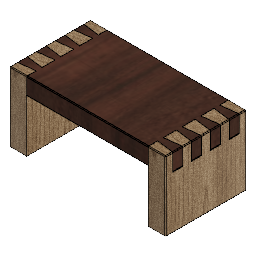
one-step-stool-dovetail (Autodesk Fusion 360 design; units mm, degrees)
Autodesk Fusion 360 part; units mm, degrees
sketch "Sketch1" plane through (0, 0, 0) normal (0, 0, 1) x (1, 0, 0) in component "Top"
  line L0 (38.1, 184.15) -> (38.1, 0) construction
  line L1 (342.9, 92.075) -> (0, 92.075) construction
  line L2 (38.1, 92.075) -> (38.1, 74.6294)
  line L3 (38.1, 74.6294) -> (0, 79.375)
  line L4 (0, 79.375) -> (0, 57.15)
  line L5 (0, 57.15) -> (38.1, 61.8956)
  line L6 (38.1, 61.8956) -> (38.1, 33.3544)
  line L7 (38.1, 33.3544) -> (0, 38.1)
  line L8 (0, 38.1) -> (0, 15.875)
  line L9 (0, 15.875) -> (38.1, 20.6206)
  line L10 (38.1, 20.6206) -> (38.1, 0)
  line L11 (0, 92.075) -> (0, 0) construction
  line L12 (38.1, 163.5294) -> (38.1, 184.15)
  line L13 (0, 168.275) -> (38.1, 163.5294)
  line L14 (0, 146.05) -> (0, 168.275)
  line L15 (38.1, 150.7956) -> (0, 146.05)
  line L16 (38.1, 122.2544) -> (38.1, 150.7956)
  line L17 (0, 127) -> (38.1, 122.2544)
  line L18 (0, 104.775) -> (0, 127)
  line L19 (38.1, 109.5206) -> (0, 104.775)
  line L20 (38.1, 92.075) -> (38.1, 109.5206)
  line L21 (171.45, 0) -> (171.45, 398.9045) construction
  line L22 (342.9, 104.775) -> (342.9, 127)
  line L23 (304.8, 92.075) -> (304.8, 109.5206)
  line L24 (342.9, 15.875) -> (304.8, 20.6206)
  line L25 (304.8, 109.5206) -> (342.9, 104.775)
  line L26 (342.9, 127) -> (304.8, 122.2544)
  line L27 (304.8, 163.5294) -> (304.8, 184.15)
  line L28 (304.8, 74.6294) -> (342.9, 79.375)
  line L29 (304.8, 92.075) -> (304.8, 74.6294)
  line L30 (304.8, 122.2544) -> (304.8, 150.7956)
  line L31 (342.9, 168.275) -> (304.8, 163.5294)
  line L32 (304.8, 33.3544) -> (342.9, 38.1)
  line L33 (304.8, 184.15) -> (304.8, 0) construction
  line L34 (304.8, 20.6206) -> (304.8, 0)
  line L35 (304.8, 61.8956) -> (304.8, 33.3544)
  line L36 (342.9, 92.075) -> (342.9, 0) construction
  line L37 (342.9, 146.05) -> (342.9, 168.275)
  line L38 (342.9, 79.375) -> (342.9, 57.15)
  line L39 (304.8, 150.7956) -> (342.9, 146.05)
  line L40 (342.9, 38.1) -> (342.9, 15.875)
  line L41 (342.9, 57.15) -> (304.8, 61.8956)
  line L42 (38.1, 184.15) -> (304.8, 184.15)
  line L43 (38.1, 0) -> (304.8, 0)
  point P0 (342.9, 0)
  dimension "d5" = 38.1
  dimension "d6" = 82.9
  dimension "d8" = 82.9
  dimension "d9" = 82.9
  dimension "d10" = 82.9
  dimension "d11" = 12.7
  dimension "d12" = 22.225
  dimension "d13" = 15.875
  dimension "d14" = 22.225
  dimension "d15" = 92.075
  dimension "d16" = 342.9
  dimension "d17" = 184.15
  constraint coincident L11.end origin
  constraint midpoint L0 L2.start
  constraint coincident L0 L2.end
  constraint coincident L0 L5.end
  constraint coincident L0 L6.end
  constraint parallel L0 L6
  constraint coincident L0 L9.end
  constraint vertical L4
  constraint vertical L8
  constraint collinear L8 L11
  constraint collinear L4 L11
  constraint symmetric L0.end L1 L0.start
  constraint symmetric L1 L2.start L20.start
  constraint symmetric L1 L2.end L19.start
  constraint symmetric L1 L3.end L18.start
  constraint symmetric L1 L4.end L17.start
  constraint symmetric L1 L5.end L16.start
  constraint symmetric L1 L6.end L15.start
  constraint symmetric L1 L7.end L14.start
  constraint symmetric L1 L8.end L13.start
  constraint symmetric L1 L9.end L12.start
  constraint symmetric L11.end L21 L36.end
  constraint symmetric L11.end L21 P0
  constraint symmetric L0.start L21 L27.end
  constraint symmetric L0.end L21 L33.end
  constraint symmetric L1.end L21 L1.start
  constraint symmetric L2.start L21 L23.start
  constraint symmetric L2.end L21 L28.start
  constraint symmetric L3.end L21 L28.end
  constraint symmetric L4.end L21 L38.end
  constraint symmetric L5.end L21 L35.start
  constraint symmetric L6.end L21 L32.start
  constraint symmetric L7.end L21 L32.end
  constraint symmetric L8.end L21 L24.start
  constraint symmetric L9.end L21 L24.end
  constraint symmetric L12.start L21 L27.start
  constraint symmetric L13.start L21 L31.start
  constraint symmetric L14.start L21 L37.start
  constraint symmetric L15.start L21 L30.end
  constraint symmetric L16.start L21 L26.end
  constraint symmetric L17.start L21 L22.end
  constraint symmetric L18.start L21 L22.start
  constraint symmetric L19.start L21 L23.end
  constraint perpendicular L27 L42
  constraint perpendicular L33 L43
  measures "d5" distance of L11.end L0.end
  measures "d6" angle of L2 L3
  measures "d8" angle of L5 L6
  measures "d9" angle of L6 L7
  measures "d10" angle of L9 L10
  measures "d11" distance of L1.end L3.end
  measures "d12" distance of L3.end L4.end
  measures "d13" distance of L11.end L8.end
  measures "d14" distance of L7.end L8.end
  measures "d15" distance of L11.end L1.end
  measures "d16" distance of L14 L37
  measures "d17" distance of L42 L43
sketch "Sketch2" plane through (0, 0, 0) normal (0, 0, 1) x (1, 0, 0) in component "Top"
  line L0 (3.0624, 88.9) -> (129.9288, 88.9) construction
  line L1 (38.1, 0) -> (38.1, 20.6206)
  line L2 (38.1, 20.6206) -> (0, 15.875)
  line L3 (0, 15.875) -> (0, 38.1)
  line L4 (0, 38.1) -> (38.1, 33.3544)
  line L5 (38.1, 33.3544) -> (38.1, 61.8956)
  line L6 (38.1, 61.8956) -> (0, 57.15)
  line L7 (0, 57.15) -> (0, 79.375)
  line L8 (0, 79.375) -> (38.1, 74.6294)
  line L9 (38.1, 74.6294) -> (38.1, 88.9)
  line L10 (38.1, 61.8956) -> (38.1, 74.6294) construction
  line L11 (0, 0) -> (101.4226, 0) construction
  line L12 (0, 0) -> (0, 254.7903) construction
  line L13 (38.1, 177.8) -> (38.1, 157.1794)
  line L14 (38.1, 157.1794) -> (0, 161.925)
  line L15 (0, 161.925) -> (0, 139.7)
  line L16 (0, 139.7) -> (38.1, 144.4456)
  line L17 (38.1, 144.4456) -> (38.1, 115.9044)
  line L18 (38.1, 115.9044) -> (0, 120.65)
  line L19 (0, 120.65) -> (0, 98.425)
  line L20 (0, 98.425) -> (38.1, 103.1706)
  line L21 (38.1, 103.1706) -> (38.1, 88.9)
  line L22 (171.45, -19.8765) -> (171.45, 334.6379) construction
  line L23 (304.8, 61.8956) -> (304.8, 74.6294) construction
  line L24 (304.8, 74.6294) -> (304.8, 88.9)
  line L25 (342.9, 38.1) -> (304.8, 33.3544)
  line L26 (342.9, 79.375) -> (304.8, 74.6294)
  line L27 (304.8, 0) -> (304.8, 20.6206)
  line L28 (342.9, 120.65) -> (342.9, 98.425)
  line L29 (304.8, 20.6206) -> (342.9, 15.875)
  line L30 (342.9, 161.925) -> (342.9, 139.7)
  line L31 (342.9, 139.7) -> (304.8, 144.4456)
  line L32 (304.8, 33.3544) -> (304.8, 61.8956)
  line L33 (304.8, 177.8) -> (304.8, 157.1794)
  line L34 (304.8, 103.1706) -> (304.8, 88.9)
  line L35 (304.8, 157.1794) -> (342.9, 161.925)
  line L36 (304.8, 115.9044) -> (342.9, 120.65)
  line L37 (342.9, 15.875) -> (342.9, 38.1)
  line L38 (342.9, 98.425) -> (304.8, 103.1706)
  line L39 (304.8, 144.4456) -> (304.8, 115.9044)
  line L40 (342.9, 57.15) -> (342.9, 79.375)
  line L41 (304.8, 61.8956) -> (342.9, 57.15)
  line L42 (38.1, 0) -> (304.8, 0)
  line L43 (38.1, 177.8) -> (304.8, 177.8)
  line L44 (342.9, 177.8) -> (0, 177.8)
  line L45 (0, 177.8) -> (0, 0)
  line L46 (0, 0) -> (342.9, 0)
  line L47 (342.9, 0) -> (342.9, 177.8)
  line L48 (0, 177.8) -> (0, 0)
  line L49 (38.1, 177.8) -> (38.1, 0)
  point P0 (342.9, 0)
  point P1 (339.8376, 88.9)
  point P2 (342.9, 0)
  point P3 (342.9, 0)
  dimension "d21" = 88.9
  dimension "d22" = 38.1
  dimension "d24" = 82.9
  dimension "d25" = 38.1
  dimension "d26" = 97.1
  dimension "d27" = 9.525
  dimension "d28" = 15.875
  dimension "d30" = 22.225
  dimension "d31" = 22.225
  dimension "d32" = 171.45
  constraint vertical L1
  constraint parallel L1 L3
  constraint parallel L4 L8
  constraint perpendicular L0 L9
  constraint parallel L2 L6
  constraint coincident L0 L9.end
  constraint coincident L11.start L12.start
  constraint perpendicular L3 L11
  constraint coincident L1.start L11
  constraint collinear L5 L9
  constraint collinear L1 L5
  constraint perpendicular L11 L12
  constraint collinear L7 L12
  constraint symmetric L0 L1.start L13.start
  constraint symmetric L0 L1.end L13.end
  constraint symmetric L0 L2.end L14.end
  constraint symmetric L0 L3.end L15.end
  constraint symmetric L0 L4.end L16.end
  constraint symmetric L0 L5.end L17.end
  constraint symmetric L0 L6.end L18.end
  constraint symmetric L0 L7.end L19.end
  constraint symmetric L0 L8.end L20.end
  constraint symmetric L0 L9.end L21.end
  constraint vertical L22
  constraint symmetric L11.start L22 P3
  constraint symmetric L0.start L22 P1
  constraint symmetric L1.start L22 L27.start
  constraint symmetric L1.end L22 L27.end
  constraint symmetric L2.end L22 L29.end
  constraint symmetric L3.end L22 L25.start
  constraint symmetric L4.end L22 L25.end
  constraint symmetric L5.end L22 L23.start
  constraint symmetric L6.end L22 L40.start
  constraint symmetric L7.end L22 L26.start
  constraint symmetric L8.end L22 L23.end
  constraint symmetric L9.end L22 L24.end
  constraint symmetric L13.start L22 L33.start
  constraint symmetric L13.end L22 L33.end
  constraint symmetric L14.end L22 L30.start
  constraint symmetric L15.end L22 L30.end
  constraint symmetric L16.end L22 L31.end
  constraint symmetric L17.end L22 L36.start
  constraint symmetric L18.end L22 L28.start
  constraint symmetric L19.end L22 L28.end
  constraint symmetric L20.end L22 L34.start
  constraint horizontal L44
  constraint vertical L45
  constraint horizontal L46
  constraint vertical L47
  constraint collinear L42 L46
  constraint collinear L15 L45
  constraint collinear L37 L47
  constraint collinear L43 L44
  measures "d21" vertical distance of L11.start L0.start
  measures "d22" distance of L1 L3
  measures "d24" angle of L8 L9
  measures "d25" horizontal distance of L7.end L9.end
  measures "d26" angle of L6 L10
  measures "d27" distance of L0 L7.end
  measures "d28" distance of L2.end L11
  measures "d30" distance of L6.end L7.end
  measures "d31" distance of L2.end L3.end
  measures "d32" distance of L12 L22
sketch "Sketch3" plane through (0, 0, 0) normal (0, 0, 1) x (1, 0, 0) in component "Top"
  line L0 (342.9, 177.8) -> (0, 177.8)
  line L1 (0, 177.8) -> (0, 0)
  line L2 (0, 0) -> (342.9, 0)
  line L3 (342.9, 0) -> (342.9, 177.8)
  dimension "d33" = 177.8
  dimension "d34" = 342.9
  constraint horizontal L0
  constraint vertical L1
  constraint horizontal L2
  constraint vertical L3
  constraint coincident L1.end L2.start
  measures "d33" distance of L0.start L2.end
  measures "d34" distance of L1.end L2.end
extrude "Extrude1" add sketch "Sketch3" along normal blind 38.1 makes body 1 in component "Top"
sketch "Sketch4" plane through (0, 0, 38.1) normal (0, 0, 1) x (-1, 0, 0) in component "Top"
  line L0 (-342.9, 0) -> (-342.9, -177.8)
  line L1 (-342.9, -177.8) -> (0, -177.8)
  line L2 (0, -177.8) -> (0, 0)
  line L3 (0, 0) -> (-342.9, 0)
  line L4 (0, -88.9) -> (-342.9, -88.9) construction
  line L5 (-171.45, -177.8) -> (-171.45, 0)
  line L6 (-38.1, -177.8) -> (-38.1, 0) construction
  line L7 (-38.1, -88.9) -> (-38.1, -74.6294)
  line L8 (-38.1, -74.6294) -> (0, -79.375)
  line L9 (0, -79.375) -> (0, -57.15)
  line L10 (0, -57.15) -> (-38.1, -61.8956)
  line L11 (-38.1, -61.8956) -> (-38.1, -33.3544)
  line L12 (-38.1, -33.3544) -> (0, -38.1)
  line L13 (0, -38.1) -> (0, -15.875)
  line L14 (0, -15.875) -> (-38.1, -20.6206)
  line L15 (-38.1, -20.6206) -> (-38.1, 0)
  line L16 (-38.1, -157.1794) -> (-38.1, -177.8)
  line L17 (0, -161.925) -> (-38.1, -157.1794)
  line L18 (0, -139.7) -> (0, -161.925)
  line L19 (-38.1, -144.4456) -> (0, -139.7)
  line L20 (-38.1, -115.9044) -> (-38.1, -144.4456)
  line L21 (0, -120.65) -> (-38.1, -115.9044)
  line L22 (0, -98.425) -> (0, -120.65)
  line L23 (-38.1, -103.1706) -> (0, -98.425)
  line L24 (-38.1, -88.9) -> (-38.1, -103.1706)
  line L25 (-304.8, -177.8) -> (-304.8, 0) construction
  line L26 (-342.9, -161.925) -> (-304.8, -157.1794)
  line L27 (-342.9, -139.7) -> (-342.9, -161.925)
  line L28 (-304.8, -144.4456) -> (-342.9, -139.7)
  line L29 (-304.8, -115.9044) -> (-304.8, -144.4456)
  line L30 (-342.9, -120.65) -> (-304.8, -115.9044)
  line L31 (-342.9, -98.425) -> (-342.9, -120.65)
  line L32 (-304.8, -103.1706) -> (-342.9, -98.425)
  line L33 (-304.8, -88.9) -> (-304.8, -103.1706)
  line L34 (-304.8, -74.6294) -> (-342.9, -79.375)
  line L35 (-342.9, -79.375) -> (-342.9, -57.15)
  line L36 (-342.9, -57.15) -> (-304.8, -61.8956)
  line L37 (-304.8, -61.8956) -> (-304.8, -33.3544)
  line L38 (-304.8, -33.3544) -> (-342.9, -38.1)
  line L39 (-342.9, -38.1) -> (-342.9, -15.875)
  line L40 (-342.9, -15.875) -> (-304.8, -20.6206)
  line L41 (-304.8, -20.6206) -> (-304.8, 0)
  line L42 (-304.8, -157.1794) -> (-304.8, -177.8)
  line L43 (-304.8, -103.1706) -> (-304.8, -74.6294)
  point P0 (-38.1, -88.9)
  dimension "d37" = 38.1
  dimension "d38" = 38.1
  dimension "d40" = 82.9
  dimension "d41" = 9.525
  dimension "d42" = 88.9
  dimension "d43" = 22.225
  dimension "d44" = 82.9
  dimension "d45" = 82.9
  dimension "d46" = 82.9
  dimension "d47" = 22.225
  dimension "d48" = 15.875
  constraint midpoint L2 L4.start
  constraint midpoint L0 L4.end
  constraint midpoint L1 L5.start
  constraint midpoint L3 L5.end
  constraint coincident L1 L6.start
  constraint coincident L3 L6.end
  constraint perpendicular L3 L6
  constraint vertical L7
  constraint vertical L11
  constraint vertical L15
  constraint vertical L9
  constraint vertical L13
  constraint collinear L7 L11
  constraint collinear L11 L15
  constraint collinear L9 L13
  constraint collinear L2 L9
  constraint midpoint L6 P0
  constraint coincident P0 L7.start
  constraint symmetric L4 P0 L7.start
  constraint symmetric L4 L7.end L23.start
  constraint symmetric L4 L8.end L22.start
  constraint symmetric L4 L9.end L21.start
  constraint symmetric L4 L10.end L20.start
  constraint symmetric L4 L11.end L19.start
  constraint symmetric L4 L12.end L18.start
  constraint symmetric L4 L13.end L17.start
  constraint symmetric L4 L14.end L16.start
  constraint symmetric L4 L6.end L6.start
  constraint symmetric L5 L6.start L25.start
  constraint symmetric L5 L6.end L25.end
  constraint symmetric L5 L7.end L34.start
  constraint symmetric L5 L8.end L34.end
  constraint symmetric L5 L9.end L35.end
  constraint symmetric L5 L10.end L36.end
  constraint symmetric L5 L11.end L37.end
  constraint symmetric L5 L12.end L38.end
  constraint symmetric L5 L13.end L39.end
  constraint symmetric L5 L14.end L40.end
  constraint symmetric L5 L16.start L26.end
  constraint symmetric L5 L17.start L26.start
  constraint symmetric L5 L18.start L27.start
  constraint symmetric L5 L19.start L28.start
  constraint symmetric L5 L20.start L29.start
  constraint symmetric L5 L21.start L30.start
  constraint symmetric L5 L22.start L31.start
  constraint symmetric L5 L23.start L32.start
  constraint symmetric L5 P0 L33.start
  measures "d37" distance of L1.end L6.start
  measures "d38" horizontal distance of P0 L8.end
  measures "d40" angle of L7 L8
  measures "d41" vertical distance of P0 L8.end
  measures "d42" distance of P0 L6.end
  measures "d43" distance of L8.end L9.end
  measures "d44" angle of L10 L11
  measures "d45" angle of L11 L12
  measures "d46" angle of L14 L15
  measures "d47" distance of L12.end L13.end
  measures "d48" vertical distance of L13.end L6.end
extrude "Extrude2" cut sketch "Sketch4" against normal through all contours L0 L3 L40 L41 | L0 L36 L37 L38 | L2 L3 L14 L15 | L0 L32 L33 L34 L43 | L0 L1 L26 L42 | L1 L2 L16 L17 | L0 L28 L29 L30 | L2 L10 L11 L12 | L2 L19 L20 L21 | L2 L7 L8 L23 L24 bodies 1 in component "Top"
sketch "Sketch5" plane through (0, 0, 38.1) normal (0, 0, 1) x (-1, 0, 0) in component "Top"
  line L0 (0, -98.425) -> (-38.1, -103.1706)
  line L1 (-38.1, -103.1706) -> (-38.1, -74.6294)
  line L2 (-38.1, -74.6294) -> (0, -79.375)
  line L3 (0, -79.375) -> (0, -57.15)
  line L4 (0, -57.15) -> (-38.1, -61.8956)
  line L5 (-38.1, -61.8956) -> (-38.1, -33.3544)
  line L6 (-38.1, -33.3544) -> (0, -38.1)
  line L7 (0, -38.1) -> (0, -15.875)
  line L8 (0, -15.875) -> (-38.1, -20.6206)
  line L9 (-38.1, -20.6206) -> (-38.1, 0)
  line L10 (-38.1, 0) -> (-304.8, 0)
  line L11 (-304.8, 0) -> (-304.8, -20.6206)
  line L12 (-304.8, -20.6206) -> (-342.9, -15.875)
  line L13 (-342.9, -15.875) -> (-342.9, -38.1)
  line L14 (-342.9, -38.1) -> (-304.8, -33.3544)
  line L15 (-304.8, -33.3544) -> (-304.8, -61.8956)
  line L16 (-304.8, -61.8956) -> (-342.9, -57.15)
  line L17 (-342.9, -57.15) -> (-342.9, -79.375)
  line L18 (-342.9, -79.375) -> (-304.8, -74.6294)
  line L19 (-304.8, -74.6294) -> (-304.8, -103.1706)
  line L20 (-304.8, -103.1706) -> (-342.9, -98.425)
  line L21 (-342.9, -98.425) -> (-342.9, -120.65)
  line L22 (-342.9, -120.65) -> (-304.8, -115.9044)
  line L23 (-304.8, -115.9044) -> (-304.8, -144.4456)
  line L24 (-304.8, -144.4456) -> (-342.9, -139.7)
  line L25 (-342.9, -139.7) -> (-342.9, -161.925)
  line L26 (-342.9, -161.925) -> (-304.8, -157.1794)
  line L27 (-304.8, -157.1794) -> (-304.8, -177.8)
  line L28 (-304.8, -177.8) -> (-38.1, -177.8)
  line L29 (-38.1, -177.8) -> (-38.1, -157.1794)
  line L30 (-38.1, -157.1794) -> (0, -161.925)
  line L31 (0, -161.925) -> (0, -139.7)
  line L32 (0, -139.7) -> (-38.1, -144.4456)
  line L33 (-38.1, -144.4456) -> (-38.1, -115.9044)
  line L34 (-38.1, -115.9044) -> (0, -120.65)
  line L35 (0, -120.65) -> (0, -98.425)
  line L36 (-38.1, -177.8) -> (0, -177.8)
  line L37 (0, -177.8) -> (0, 0)
  line L38 (0, 0) -> (-38.1, 0)
  line L39 (-38.1, 0) -> (-38.1, -177.8)
  line L40 (-304.8, -177.8) -> (-342.9, -177.8)
  line L41 (-342.9, -177.8) -> (-342.9, 0)
  line L42 (-342.9, 0) -> (-304.8, 0)
  line L43 (-304.8, 0) -> (-304.8, -177.8)
  constraint horizontal L36
  constraint vertical L37
  constraint horizontal L38
  constraint vertical L39
  constraint coincident L37.end L38.start
  constraint coincident L28.end L29.start
  constraint horizontal L40
  constraint vertical L41
  constraint horizontal L42
  constraint vertical L43
  constraint collinear L27 L43
  constraint collinear L25 L41
  constraint collinear L10 L42
  constraint collinear L28 L40
extrude "Extrude1'" add sketch "Sketch5" against normal blind 152.4 separate body contours L0 L34 L35 L37 L39 | L0 L1 L2 L37 L39 | L32 L33 L34 L37 L39 | L2 L3 L4 L37 L39 | L30 L31 L32 L37 L39 | L4 L5 L6 L37 L39 | L29 L30 L36 L37 L39 | L6 L7 L8 L37 L39 | L8 L9 L37 L38 L39 makes body 2 in component "Left"
extrude "Extrude1''" add sketch "Sketch5" against normal blind 152.4 separate body contours L26 L27 L40 L41 L43 | L11 L12 L41 L42 L43 | L24 L25 L26 L41 L43 | L12 L13 L14 L41 L43 | L22 L23 L24 L41 L43 | L14 L15 L16 L41 L43 | L20 L21 L22 L41 L43 | L16 L17 L18 L41 L43 | L18 L19 L20 L41 L43 makes body 3 in component "Right"
combine "Combine1" operation cut target body 2 tool bodies 1 keep tools in component "Left"
combine "Combine1'" operation cut target body 3 tool bodies 1 keep tools in component "Right"
chamfer "Chamfer1" distance 1.5875 angle 45 20 edges at (171.45, 0, 38.1) (171.45, 0, 0) (342.9, 68.2625, 38.1) (342.9, 109.5375, 38.1) (342.9, 26.9875, 38.1) (342.9, 150.8125, 38.1) (342.9, 150.8125, 0) (342.9, 68.2625, 0) (342.9, 109.5375, 0) (342.9, 26.9875, 0) (171.45, 177.8, 38.1) (171.45, 177.8, 0) (0, 109.5375, 38.1) (0, 68.2625, 38.1) (0, 26.9875, 38.1) (0, 150.8125, 38.1) (0, 26.9875, 0) (0, 109.5375, 0) (0, 68.2625, 0) (0, 150.8125, 0) on bodies 1 in component "Top"
chamfer "Chamfer2" distance 1.5875 angle 45 9 edges at (342.9, 0, -38.1) (342.9, 7.9375, 38.1) (342.9, 47.625, 38.1) (342.9, 88.9, 38.1) (342.9, 130.175, 38.1) (342.9, 169.8625, 38.1) (342.9, 177.8, -38.1) (323.85, 177.8, 38.1) (323.85, 0, 38.1) on bodies 3 in component "Right"
chamfer "Chamfer5" distance 1.5875 angle 45 9 edges at (19.05, 177.8, 38.1) (0, 177.8, -38.1) (0, 169.8625, 38.1) (0, 130.175, 38.1) (0, 88.9, 38.1) (0, 47.625, 38.1) (0, 7.9375, 38.1) (19.05, 0, 38.1) (0, 0, -38.1) on bodies 2 in component "Left"
component "Top" placed x (1, 0, 0) y (0, 1, 0) z (0, 0, 1) at (0, 0, 0)
component "Left" placed x (1, 0, 0) y (0, 1, 0) z (0, 0, 1) at (0, 0, 0)
component "Right" placed x (1, 0, 0) y (0, 1, 0) z (0, 0, 1) at (0, 0, 0)
equation "material_thickness = 1.5 in"
equation "d5 = material_thickness"
equation "d6 = 90 deg - dovetail_angle"
equation "dovetail_angle = 7.1 deg"
equation "d8 = 90 deg - dovetail_angle"
equation "d9 = 90 deg - dovetail_angle"
equation "d10 = 90 deg - dovetail_angle"
equation "d12 = ( 7 / 8 ) * 1 in"
equation "d13 = ( 5 / 8 ) * 1 in"
equation "d14 = d12"
equation "d21 = ( 7 / 2 ) * 1 in"
equation "d22 = material_thickness"
equation "d24 = 90 deg - dovetail_angle"
equation "d26 = 90 deg + dovetail_angle"
equation "d27 = ( 3 / 8 ) * 1 in"
equation "d28 = ( 5 / 8 ) * 1 in"
equation "d30 = ( 7 / 8 ) * 1 in"
equation "d31 = d30"
equation "d32 = ( 13.5 / 2 ) * 1 in"
equation "d35 = material_thickness"
equation "d37 = material_thickness"
equation "d38 = material_thickness"
equation "d40 = 90 deg - dovetail_angle"
equation "d44 = 90 deg - dovetail_angle"
equation "d45 = d44"
equation "d46 = d45"
equation "d47 = d43"
equation "d54 = chamfer_amt"
equation "chamfer_amt = 0.0625 in"
equation "d61 = chamfer_amt"
equation "d62 = chamfer_amt"
